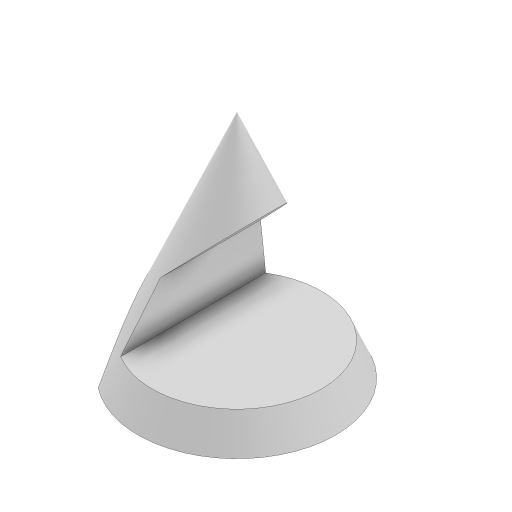
# Autodesk Inventor part: Деталь1
Saved by Autodesk Inventor 2023.2 (Build 272271030, 271C)
## iProperties
Created: 2023-10-27
Part Number: Деталь1
Material: Типовые
Document SubType Name: Modeling
Designer: User
Density: 1 g/cm^3
Appearance: По умолчанию
Author: User
Autodesk Inventor part; units mm, degrees
ref_plane "YZ Plane" through (0, 0, 0) normal (1, 0, 0) x (0, 1, 0)
ref_plane "XZ Plane" through (0, 0, 0) normal (0, 1, 0) x (-1, 0, 0)
ref_plane "XY Plane" through (0, 0, 0) normal (0, 0, 1) x (1, 0, 0)
sketch "Эскиз1" plane through (0, 0, 0) normal (1, 0, 0) x (0, 1, 0)
  line L0 (70, 0) -> (0, 0)
  line L1 (0, 0) -> (0, -30)
  line L2 (0, -30) -> (70, 0)
  dimension "d0" = 30
  dimension "d1" = 70
  constraints: 6 end point, 1 horizontal, 1 perpendicular
  measures "d0" distance of L0.end L1.end
  measures "d1" distance of L0.start L0.end
revolve "Вращение1" add sketch "Эскиз1" angle 360 about axis through (0, 70, 0) along (0, -1, 0)
sketch "Эскиз2" plane through (0, 0, 0) normal (0, 0, 1) x (1, 0, 0)
  line L0 (0, 70) -> (30, 0) projected
  line L1 (25.7143, 10) -> (-13.2857, 10)
  line L2 (-30, 0) -> (30, 0) projected
  line L3 (-8, 30) -> (-13.2857, 10)
  line L4 (-8, 30) -> (9.4286, 48)
  line L5 (-18.3924, 0) -> (-18.3924, 27.0844)
  line L6 (0, 70) -> (-30, 0) projected
  point P0 (0, 0)
  point P1 (0, 30)
  constraints: 8 end point, 4 point on line, 1 horizontal
extrude "Выдавливание1" cut sketch "Эскиз2" along normal mid plane 100 contours L0 L1 L3 L4 | L5 L2 L6
